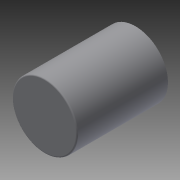
# Autodesk Inventor part: Outer Layer
Saved by Autodesk Inventor 2015 (Build 190159000, 159)
## iProperties
Created: 2018-04-06
Part Number: Outer Layer
Material: Generic
Document SubType Name: Modeling
Designer: Administrator
Density: 1 g/cm^3
Appearance: Default
Author: Administrator
Autodesk Inventor part; units mm, degrees
ref_plane "YZ Plane" through (0, 0, 0) normal (1, 0, 0) x (0, 1, 0)
ref_plane "XZ Plane" through (0, 0, 0) normal (0, 1, 0) x (-1, 0, 0)
ref_plane "XY Plane" through (0, 0, 0) normal (0, 0, 1) x (1, 0, 0)
sketch "Sketch1" plane through (0, 0, 0) normal (0, 1, 0) x (-1, 0, 0)
  circle A0 centre (0, 0) radius 50
  dimension "d0" = 100
  constraints: 1 centre point, 1 coincident
  measures "d0" diameter of A0
extrude "Extrusion1" add sketch "Sketch1" along normal blind 140
shell "Shell1" thickness 5 removed faces 1 at (-9.39, 140, -8.8667)
fillet "Fillet1" radius 2 2 edges at (50, 0, 0) (45, 5, 0)
body "Solid1"
